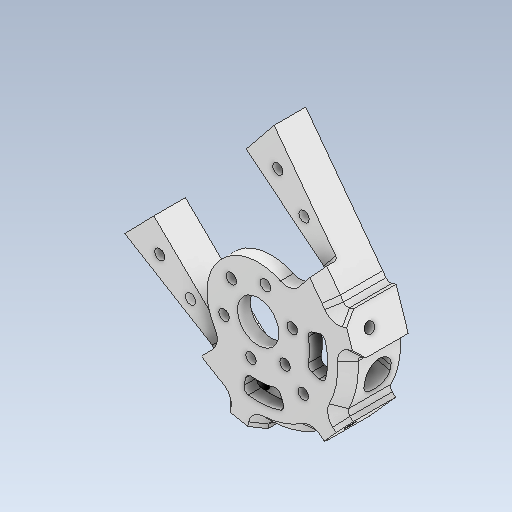
# Autodesk Inventor part: end_holder_1
Saved by Autodesk Inventor 2020 (Build 240168000, 168)
## iProperties
Created: 2020-08-12
Part Number: end_holder_1
Material: ABS Plastic
Document SubType Name: Modeling
Designer: psrobotics
Density: 1.06 g/cm^3
Appearance: Smooth - White
Author: psrobotics
Autodesk Inventor part; units mm, degrees
(part 1 of 2)
ref_plane "Work Plane1" through (0, 0, 1) normal (0, 0, 1) x (1, 0, 0)
sketch "Sketch1" plane through (0, 0, 1) normal (0, 0, 1) x (1, 0, 0)
  arc A0 (-18.1219, -29.9432) -> (28.0322, 20.957) centre (0, 0) ccw projected
  circle A1 centre (0, 0) radius 35
  circle A2 centre (0, 0) radius 26.3 projected
  circle A3 centre (0, 0) radius 29
  point P0 (0, 0)
  point P1 (28.0322, 20.957)
  dimension "d0" = 70
  dimension "d1" = 58
  constraints: 2 centre point, 2 coincident
  measures "d0" diameter of A1
  measures "d1" diameter of A3
ref_plane "Work Plane2" through (-254.295, -122.3855, -14.5) normal (0, 0, 1) x (0.9725249, -0.2327991, 0)
extrude "Extrusion1" add sketch "Sketch1" against normal up to surface (15.5 mm away) contours A1 A0
sketch "Sketch2" plane through (0, 0, 1) normal (0, 0, 1) x (1, 0, 0)
  circle A0 centre (-84.1417, 77.6558) radius 21 projected
  arc A1 (22.0166, 27.2079) -> (-24.4063, -25.0865) centre (0, 0) ccw projected
  line L0 (22.0166, 27.2079) -> (-113.9368, 137.2214) projected
  line L1 (-113.9368, 137.2214) -> (-123.7838, 141.4952) projected
  arc A2 (-156.6916, 110.1172) -> (-123.7838, 141.4952) centre (-169.0182, 155.9899) ccw projected
  line L2 (-156.6916, 110.1172) -> (-153.0652, 100.0837) projected
  line L3 (-153.0652, 100.0837) -> (-24.4063, -25.0865) projected
  circle A3 centre (-131.7071, 116.2642) radius 1.55 projected
  circle A4 centre (-150.4931, 104.7349) radius 1.55 projected
  circle A5 centre (-119.024, 134.2913) radius 1.55 projected
  circle A6 centre (0, 0) radius 35 projected
  circle A7 centre (0, 0) radius 29 projected
  line L4 (0, 0) -> (-24.4063, -25.0865)
  line L5 (0, 0) -> (22.0166, 27.2079)
  circle A8 centre (0, 0) radius 29 projected
  line L6 (-20.2223, -20.786) -> (-48.8927, 7.1069)
  line L7 (18.2423, 22.5437) -> (-12.8524, 47.7055)
  line L8 (-48.8927, 7.1069) -> (-53.0766, 2.8064)
  line L9 (-12.8524, 47.7055) -> (-9.0781, 52.3697)
  point P0 (0, 0)
  point P1 (3.0091, 34.8704)
  point P2 (-34.2679, -7.1213)
  dimension "d4" = 40
  dimension "d5" = 40
  constraints: 12 end point, 4 perpendicular, 4 point on line, 2 point on circle, 2 tangent
  measures "d4" distance of L6.start L6.end
  measures "d5" distance of L7.start L7.end
ref_plane "Work Plane3" through (-254.295, -122.3855, -14.5) normal (0, 0, 1) x (0.9725249, -0.2327991, 0)
extrude "Extrusion2" add sketch "Sketch2" against normal up to surface (15.5 mm away) contours A1 L7 L9 L0 | A1 L3 L8 L6
sketch "Sketch3" plane through (0, 0, 1) normal (0, 0, 1) x (1, 0, 0)
  arc A0 (-24.4063, -25.0865) -> (22.0166, 27.2079) centre (0, 0) ccw projected
  line L0 (22.0166, 27.2079) -> (-9.0781, 52.3697) projected
  line L1 (-9.0781, 52.3697) -> (-12.8524, 47.7055) projected
  line L2 (-12.8524, 47.7055) -> (3.0091, 34.8704) projected
  arc A1 (3.0091, 34.8704) -> (-34.2679, -7.1213) centre (0, 0) ccw projected
  line L3 (-34.2679, -7.1213) -> (-48.8927, 7.1069) projected
  line L4 (-48.8927, 7.1069) -> (-53.0766, 2.8064) projected
  line L5 (-53.0766, 2.8064) -> (-24.4063, -25.0865) projected
  circle A2 centre (0, 0) radius 29 projected
  line L6 (-34.2679, -7.1213) -> (-20.2223, -20.786)
  circle A3 centre (0, 0) radius 29 projected
  line L7 (3.0091, 34.8704) -> (18.2423, 22.5437)
  point P0 (0, 0)
  point P1 (-20.2223, -20.786)
  point P2 (18.2423, 22.5437)
  constraints: 4 end point, 2 point on circle, 2 tangent
ref_plane "Work Plane4" through (-254.295, -122.3855, -14.5) normal (0, 0, 1) x (0.9725249, -0.2327991, 0)
extrude "Extrusion3" cut sketch "Sketch3" against normal up to surface (15.5 mm away) contours A1 L7 A2 L6
sketch "Sketch4" plane through (0, 0, 1) normal (0, 0, 1) x (1, 0, 0)
  circle A0 centre (0, 0) radius 22 projected
  arc A1 (-134.634, 104.1043) -> (-137.4986, 97.7068) centre (-84.1417, 77.6558) ccw projected
  arc A2 (-140.9928, 97.2403) -> (-137.4986, 97.7068) centre (-139.3708, 98.4103) ccw projected
  arc A3 (-140.9928, 97.2403) -> (-143.7017, 100.0363) centre (-151.9418, 89.3428) ccw projected
  arc A4 (-143.3582, 103.4179) -> (-143.7017, 100.0363) centre (-142.481, 101.6206) ccw projected
  arc A5 (-143.3582, 103.4179) -> (-137.4838, 106.7169) centre (-169.0182, 155.9899) ccw projected
  arc A6 (-134.634, 104.1043) -> (-137.4838, 106.7169) centre (-136.4057, 105.0323) ccw projected
  arc A7 (-141.6259, 76.3096) -> (-139.9648, 63.8706) centre (-84.1417, 77.6558) ccw projected
  arc A8 (-143.4147, 62.0777) -> (-139.9648, 63.8706) centre (-141.9064, 63.3911) ccw projected
  line L0 (-143.4147, 62.0777) -> (-152.5393, 72.5562) projected
  arc A9 (-151.1485, 75.8661) -> (-152.5393, 72.5562) centre (-151.031, 73.8696) ccw projected
  arc A10 (-151.1485, 75.8661) -> (-144.6984, 77.9505) centre (-151.9418, 89.3428) ccw projected
  arc A11 (-141.6259, 76.3096) -> (-144.6984, 77.9505) centre (-143.6254, 76.2628) ccw projected
  arc A12 (-172.9205, 88.3973) -> (-165.3006, 73.1397) centre (-151.9418, 89.3428) ccw projected
  arc A13 (-170.8017, 90.4837) -> (-172.9205, 88.3973) centre (-170.9225, 88.4874) ccw projected
  line L1 (-170.8017, 90.4837) -> (-167.2842, 90.2709) projected
  arc A14 (-165.4097, 88.4124) -> (-167.2842, 90.2709) centre (-167.4049, 88.2746) ccw projected
  arc A15 (-165.4097, 88.4124) -> (-160.7764, 79.135) centre (-151.9418, 89.3428) ccw projected
  arc A16 (-160.4168, 76.52) -> (-160.7764, 79.135) centre (-162.0853, 77.6227) ccw projected
  line L2 (-160.4168, 76.52) -> (-162.3598, 73.5801) projected
  arc A17 (-165.3006, 73.1397) -> (-162.3598, 73.5801) centre (-164.0284, 74.6828) ccw projected
  arc A18 (-121.303, 49.7044) -> (-115.1167, 42.9745) centre (-84.1417, 77.6558) ccw projected
  arc A19 (-120.5392, 54.0239) -> (-121.303, 49.7044) centre (-118.9055, 51.5077) ccw projected
  line L3 (-120.5392, 54.0239) -> (-118.8576, 55.1157) projected
  arc A20 (-114.8324, 54.4108) -> (-118.8576, 55.1157) centre (-117.2239, 52.5995) ccw projected
  arc A21 (-114.8324, 54.4108) -> (-109.9637, 49.0993) centre (-84.1417, 77.6558) ccw projected
  arc A22 (-109.5035, 45.1747) -> (-109.9637, 49.0993) centre (-111.9758, 46.8741) ccw projected
  line L4 (-109.5035, 45.1747) -> (-110.6461, 43.5126) projected
  arc A23 (-115.1167, 42.9745) -> (-110.6461, 43.5126) centre (-113.1183, 45.212) ccw projected
  arc A24 (-66.7292, 111.9932) -> (-73.4322, 114.6363) centre (-84.1417, 77.6558) ccw projected
  arc A25 (-75.5321, 118.142) -> (-73.4322, 114.6363) centre (-72.5977, 117.5179) ccw projected
  line L5 (-75.5321, 118.142) -> (-74.177, 124.5142) projected
  arc A26 (-70.4364, 126.7798) -> (-74.177, 124.5142) centre (-71.2426, 123.8902) ccw projected
  arc A27 (-60.257, 122.7171) -> (-70.4364, 126.7798) centre (-84.1417, 77.6558) ccw projected
  arc A28 (-59.1897, 118.367) -> (-60.257, 122.7171) centre (-61.662, 120.0665) ccw projected
  line L6 (-59.1897, 118.367) -> (-62.9002, 112.9694) projected
  arc A29 (-66.7292, 111.9932) -> (-62.9002, 112.9694) centre (-65.3724, 114.6689) ccw projected
  arc A30 (-78.2994, 26.9916) -> (-67.6092, 29.4098) centre (-84.1417, 77.6558) ccw projected
  arc A31 (-81.6389, 29.8151) -> (-78.2994, 26.9916) centre (-78.643, 29.9718) ccw projected
  line L7 (-81.6389, 29.8151) -> (-81.9793, 36.3209) projected
  arc A32 (-79.3563, 39.4544) -> (-81.9793, 36.3209) centre (-78.9834, 36.4777) ccw projected
  arc A33 (-79.3563, 39.4544) -> (-72.322, 41.0151) centre (-84.1417, 77.6558) ccw projected
  arc A34 (-68.6931, 39.4512) -> (-72.322, 41.0151) centre (-71.401, 38.16) ccw projected
  line L8 (-68.6931, 39.4512) -> (-65.8738, 33.5391) projected
  arc A35 (-67.6092, 29.4098) -> (-65.8738, 33.5391) centre (-68.5817, 32.2478) ccw projected
  arc A36 (-122.585, 75.5668) -> (-121.5224, 68.4402) centre (-84.1417, 77.6558) ccw projected
  arc A37 (-123.5085, 64.8689) -> (-121.5224, 68.4402) centre (-124.4352, 67.7221) ccw projected
  line L9 (-123.5085, 64.8689) -> (-129.7045, 62.8563) projected
  arc A38 (-133.5369, 64.9629) -> (-129.7045, 62.8563) centre (-130.6313, 65.7096) ccw projected
  arc A39 (-135.1083, 75.8099) -> (-133.5369, 64.9629) centre (-84.1417, 77.6558) ccw projected
  arc A40 (-131.8746, 78.9093) -> (-135.1083, 75.8099) centre (-132.1102, 75.9185) ccw projected
  line L10 (-131.8746, 78.9093) -> (-125.3449, 78.3947) projected
  arc A41 (-122.585, 75.5668) -> (-125.3449, 78.3947) centre (-125.5805, 75.404) ccw projected
  arc A42 (-89.984, 128.3201) -> (-100.6741, 125.9019) centre (-84.1417, 77.6558) ccw projected
  arc A43 (-86.6444, 125.4966) -> (-89.984, 128.3201) centre (-89.6403, 125.3399) ccw projected
  line L11 (-86.6444, 125.4966) -> (-86.3041, 118.9907) projected
  arc A44 (-88.9271, 115.8573) -> (-86.3041, 118.9907) centre (-89.3, 118.834) ccw projected
  arc A45 (-88.9271, 115.8573) -> (-95.9613, 114.2966) centre (-84.1417, 77.6558) ccw projected
  arc A46 (-99.5902, 115.8604) -> (-95.9613, 114.2966) centre (-96.8824, 117.1517) ccw projected
  line L12 (-99.5902, 115.8604) -> (-102.4095, 121.7726) projected
  arc A47 (-100.6741, 125.9019) -> (-102.4095, 121.7726) centre (-99.7016, 123.0639) ccw projected
  arc A48 (-41.3543, 59.4489) -> (-38.6192, 68.1713) centre (-84.1417, 77.6558) ccw projected
  arc A49 (-45.477, 57.9506) -> (-41.3543, 59.4489) centre (-44.1148, 60.6235) ccw projected
  line L13 (-45.477, 57.9506) -> (-47.2634, 58.8611) projected
  arc A50 (-48.6656, 62.6994) -> (-47.2634, 58.8611) centre (-45.9012, 61.534) ccw projected
  arc A51 (-48.6656, 62.6994) -> (-46.5, 69.5716) centre (-84.1417, 77.6558) ccw projected
  arc A52 (-43.3312, 71.9324) -> (-46.5, 69.5716) centre (-43.5669, 68.9417) ccw projected
  line L14 (-43.3312, 71.9324) -> (-41.3205, 71.7739) projected
  arc A53 (-38.6192, 68.1713) -> (-41.3205, 71.7739) centre (-41.5561, 68.7832) ccw projected
  line L15 (-106.5258, 40.6801) -> (-105.3832, 42.3423) projected
  arc A54 (-101.5541, 43.3185) -> (-105.3832, 42.3423) centre (-102.911, 40.6428) ccw projected
  arc A55 (-101.5541, 43.3185) -> (-94.8511, 40.6753) centre (-84.1417, 77.6558) ccw projected
  arc A56 (-92.7512, 37.1697) -> (-94.8511, 40.6753) centre (-95.6856, 37.7937) ccw projected
  line L16 (-92.7512, 37.1697) -> (-93.1683, 35.2086) projected
  arc A57 (-96.9276, 32.9482) -> (-93.1683, 35.2086) centre (-96.1027, 35.8326) ccw projected
  arc A58 (-105.4268, 36.3134) -> (-96.9276, 32.9482) centre (-84.1417, 77.6558) ccw projected
  arc A59 (-106.5258, 40.6801) -> (-105.4268, 36.3134) centre (-104.0535, 38.9807) ccw projected
  arc A60 (-58.7798, 110.137) -> (-58.3197, 106.2124) centre (-56.3076, 108.4375) ccw projected
  line L17 (-58.7798, 110.137) -> (-55.0694, 115.5346) projected
  arc A61 (-50.6256, 116.0964) -> (-55.0694, 115.5346) centre (-52.5971, 113.8352) ccw projected
  arc A62 (-43.1863, 108.0475) -> (-50.6256, 116.0964) centre (-84.1417, 77.6558) ccw projected
  arc A63 (-43.9617, 103.7436) -> (-43.1863, 108.0475) centre (-45.5954, 106.2598) ccw projected
  line L18 (-43.9617, 103.7436) -> (-49.4258, 100.196) projected
  arc A64 (-53.451, 100.9008) -> (-49.4258, 100.196) centre (-51.0595, 102.7121) ccw projected
  arc A65 (-53.451, 100.9008) -> (-58.3197, 106.2124) centre (-84.1417, 77.6558) ccw projected
  line L19 (-61.3607, 35.6912) -> (-64.18, 41.6034) projected
  arc A66 (-63.1109, 45.4075) -> (-64.18, 41.6034) centre (-61.4721, 42.8946) ccw projected
  arc A67 (-63.1109, 45.4075) -> (-57.4703, 49.8909) centre (-84.1417, 77.6558) ccw projected
  arc A68 (-53.3844, 49.9567) -> (-57.4703, 49.8909) centre (-55.392, 47.7274) ccw projected
  line L20 (-53.3844, 49.9567) -> (-48.5435, 45.597) projected
  arc A69 (-48.4517, 41.2248) -> (-48.5435, 45.597) centre (-50.5511, 43.3678) ccw projected
  arc A70 (-57.0598, 34.4404) -> (-48.4517, 41.2248) centre (-84.1417, 77.6558) ccw projected
  arc A71 (-61.3607, 35.6912) -> (-57.0598, 34.4404) centre (-58.6528, 36.9825) ccw projected
  arc A72 (-124.9521, 83.3793) -> (-121.7833, 85.7401) centre (-124.7165, 86.37) ccw projected
  line L21 (-124.9521, 83.3793) -> (-131.4818, 83.8938) projected
  arc A73 (-134.1902, 87.4613) -> (-131.4818, 83.8938) centre (-131.2461, 86.8845) ccw projected
  arc A74 (-130.9394, 97.9284) -> (-134.1902, 87.4613) centre (-84.1417, 77.6558) ccw projected
  arc A75 (-126.8243, 99.4088) -> (-130.9394, 97.9284) centre (-128.1866, 96.7359) ccw projected
  line L22 (-126.8243, 99.4088) -> (-121.0199, 96.4506) projected
  arc A76 (-119.6178, 92.6123) -> (-121.0199, 96.4506) centre (-122.3822, 93.7777) ccw projected
  arc A77 (-119.6178, 92.6123) -> (-121.7833, 85.7401) centre (-84.1417, 77.6558) ccw projected
  line L23 (-106.9226, 119.6204) -> (-104.1034, 113.7083) projected
  arc A78 (-105.1725, 109.9042) -> (-104.1034, 113.7083) centre (-106.8112, 112.417) ccw projected
  arc A79 (-105.1725, 109.9042) -> (-110.813, 105.4207) centre (-84.1417, 77.6558) ccw projected
  arc A80 (-114.8989, 105.355) -> (-110.813, 105.4207) centre (-112.8913, 107.5842) ccw projected
  line L24 (-114.8989, 105.355) -> (-119.7399, 109.7147) projected
  arc A81 (-119.8317, 114.0869) -> (-119.7399, 109.7147) centre (-117.7323, 111.9439) ccw projected
  arc A82 (-111.2236, 120.8712) -> (-119.8317, 114.0869) centre (-84.1417, 77.6558) ccw projected
  arc A83 (-106.9226, 119.6204) -> (-111.2236, 120.8712) centre (-109.6305, 118.3292) ccw projected
  line L25 (-40.9277, 76.7585) -> (-42.9385, 76.9169) projected
  arc A84 (-45.6984, 79.7449) -> (-42.9385, 76.9169) centre (-42.7028, 79.9077) ccw projected
  arc A85 (-45.6984, 79.7449) -> (-46.7609, 86.8714) centre (-84.1417, 77.6558) ccw projected
  arc A86 (-44.7749, 90.4428) -> (-46.7609, 86.8714) centre (-43.8481, 87.5895) ccw projected
  line L26 (-44.7749, 90.4428) -> (-42.868, 91.0622) projected
  arc A87 (-39.0308, 88.9367) -> (-42.868, 91.0622) centre (-41.9412, 88.2089) ccw projected
  arc A88 (-37.6955, 79.8936) -> (-39.0308, 88.9367) centre (-84.1417, 77.6558) ccw projected
  arc A89 (-40.9277, 76.7585) -> (-37.6955, 79.8936) centre (-40.6921, 79.7492) ccw projected
  circle A90 centre (-150.4931, 104.7349) radius 2.1 projected
  circle A91 centre (-131.7071, 116.2642) radius 2.1 projected
  circle A92 centre (-172.3092, 101.5894) radius 2.1 projected
  circle A93 centre (-119.024, 134.2913) radius 2.1 projected
  circle A94 centre (-151.9418, 89.3428) radius 8 projected
  line L27 (-121.4797, 140.4951) -> (-109.1576, 143.9934) projected
  arc A95 (-172.0375, 106.0811) -> (-121.4797, 140.4951) centre (-169.0182, 155.9899) ccw projected
  line L28 (-172.0375, 106.0811) -> (-180.4523, 106.5902) projected
  line L29 (-180.4523, 106.5902) -> (-181.871, 83.1388) projected
  line L30 (-181.871, 83.1388) -> (-178.1654, 82.9146) projected
  arc A96 (-178.1654, 82.9146) -> (-161.4844, 64.0853) centre (-151.9418, 89.3428) ccw projected
  line L31 (-161.4844, 64.0853) -> (-161.7085, 60.3797) projected
  line L32 (-161.7085, 60.3797) -> (-153.7231, 59.8966) projected
  line L33 (-153.7231, 59.8966) -> (-113.0893, 33.8576) projected
  line L34 (-113.0893, 33.8576) -> (-116.9889, 27.9573) projected
  line L35 (-116.9889, 27.9573) -> (-102.5081, 21.1281) projected
  line L36 (-102.5081, 21.1281) -> (-18.1219, -29.9432) projected
  arc A97 (-18.1219, -29.9432) -> (28.0322, 20.957) centre (0, 0) ccw projected
  line L37 (28.0322, 20.957) -> (-27.0336, 94.6133) projected
  line L38 (-27.0336, 94.6133) -> (-33.7368, 109.1529) projected
  arc A98 (-33.7368, 109.1529) -> (-36.6738, 113.4261) centre (-84.1417, 77.6558) ccw projected
  line L39 (-36.6738, 113.4261) -> (-37.4491, 112.8418) projected
  arc A99 (-40.2079, 113.1815) -> (-37.4491, 112.8418) centre (-38.6527, 114.4391) ccw projected
  arc A100 (-40.2079, 113.1815) -> (-46.2045, 119.5249) centre (-84.1417, 77.6558) ccw projected
  arc A101 (-46.3887, 122.2985) -> (-46.2045, 119.5249) centre (-44.8616, 121.007) ccw projected
  line L40 (-46.3887, 122.2985) -> (-45.5261, 123.3186) projected
  arc A102 (-45.5261, 123.3186) -> (-50.5107, 127.1049) centre (-84.1417, 77.6558) ccw projected
  line L41 (-50.5107, 127.1049) -> (-61.0603, 132.8238) projected
  arc A103 (-61.0603, 132.8238) -> (-66.9533, 134.9342) centre (-84.1417, 77.6558) ccw projected
  line L42 (-66.9533, 134.9342) -> (-67.3373, 133.6546) projected
  arc A104 (-69.762, 132.2953) -> (-67.3373, 133.6546) centre (-69.2529, 134.2295) ccw projected
  arc A105 (-69.762, 132.2953) -> (-78.35, 133.8582) centre (-84.1417, 77.6558) ccw projected
  arc A106 (-80.1403, 135.9846) -> (-78.35, 133.8582) centre (-78.145, 135.8477) ccw projected
  line L43 (-80.1403, 135.9846) -> (-80.0739, 136.9531) projected
  arc A107 (-80.0739, 136.9531) -> (-85.2575, 137.082) centre (-84.1417, 77.6558) ccw projected
  line L44 (-85.2575, 137.082) -> (-101.0991, 134.7639) projected
  line L45 (-101.0991, 134.7639) -> (-109.1576, 143.9934) projected
  circle A108 centre (-178.1359, 86.9201) radius 1.5 projected
  circle A109 centre (-100.501, 24.1648) radius 1.5 projected
  circle A110 centre (-64.7276, 24.8072) radius 1.5 projected
  circle A111 centre (-37.2263, 108.1168) radius 1.5 projected
  circle A112 centre (-65.0433, 130.6194) radius 1.5 projected
  circle A113 centre (-84.2213, 133.5925) radius 1.5 projected
  circle A114 centre (-50.1841, 122.5643) radius 1.5 projected
  circle A115 centre (-48.1253, 34.857) radius 1.5 projected
  circle A116 centre (-81.2881, 21.4264) radius 1.5 projected
  circle A117 centre (-157.5045, 63.6318) radius 1.5 projected
  circle A118 centre (-84.1417, 77.6558) radius 32.5 projected
  line L46 (-20.2223, -20.786) -> (-48.8927, 7.1069) projected
  line L47 (-48.8927, 7.1069) -> (-53.0766, 2.8064) projected
  line L48 (-53.0766, 2.8064) -> (-24.4063, -25.0865) projected
  arc A119 (-24.4063, -25.0865) -> (22.0166, 27.2079) centre (0, 0) ccw projected
  line L49 (22.0166, 27.2079) -> (-9.0781, 52.3697) projected
  line L50 (-9.0781, 52.3697) -> (-12.8524, 47.7055) projected
  line L51 (-12.8524, 47.7055) -> (18.2423, 22.5437) projected
  arc A120 (-20.2223, -20.786) -> (18.2423, 22.5437) centre (0, 0) ccw projected
  line L52 (-12.8524, 47.7055) -> (-9.0781, 52.3697) projected
  line L53 (-9.0781, 52.3697) -> (-1.9955, 61.1223)
  line L54 (-53.0766, 2.8064) -> (-60.1765, -4.4914)
  line L55 (-48.8927, 7.1069) -> (-53.0766, 2.8064) projected
  circle A121 centre (9.6755, 36.1764) radius 2 projected
  circle A122 centre (-34.5876, -13.7627) radius 2 projected
  circle A123 centre (-0.5842, 47.1189) radius 2 projected
  circle A124 centre (-46.5558, -4.7204) radius 2 projected
  point P0 (0, 0)
  point P1 (-18.1219, -29.9432)
  point P2 (28.0322, 20.957)
  constraints: 4 end point, 3 point on line, 1 collinear
extrude "Extrusion4" add sketch "Sketch4" against normal up to surface (15.5 mm away) contours L54 L48 A124 A122 A119 L36 | A119 L49 A121 A123 L53 L37 | L48 A124 | A122 L48 | L49 A121 | A123 L49 picked at (-46.2816, -4.9711) picked at (-35.4873, -14.8787) picked at (9.9892, 37.2529) picked at (-0.3031, 46.513)
ref_plane "Work Plane5" through (-227.4633, -98.5759, -2.2) normal (0, 0, -1) x (0.2327991, 0.9725249, 0)
sketch "Sketch5" plane through (0, 0, 1) normal (0, 0, 1) x (1, 0, 0)
  line L0 (-20.2223, -20.786) -> (-48.8927, 7.1069) projected
  line L1 (-48.8927, 7.1069) -> (-60.1765, -4.4914) projected
  line L2 (-60.1765, -4.4914) -> (-18.1219, -29.9432) projected
  arc A0 (-18.1219, -29.9432) -> (28.0322, 20.957) centre (0, 0) ccw projected
  line L3 (28.0322, 20.957) -> (-1.9955, 61.1223) projected
  line L4 (-1.9955, 61.1223) -> (-12.8524, 47.7055) projected
  line L5 (-12.8524, 47.7055) -> (18.2423, 22.5437) projected
  arc A1 (-20.2223, -20.786) -> (18.2423, 22.5437) centre (0, 0) ccw projected
  line L6 (-60.1765, -4.4914) -> (-18.1219, -29.9432) projected
  line L7 (0, 0) -> (-18.1219, -29.9432)
  line L8 (28.0322, 20.957) -> (-1.9955, 61.1223) projected
  line L9 (0, 0) -> (28.0322, 20.957)
  point P0 (0, 0)
  point P1 (23.2267, 17.3644)
  point P2 (-15.0153, -24.8101)
  constraints: 4 end point, 2 perpendicular
extrude "Extrusion5" cut sketch "Sketch5" against normal up to surface (3.2 mm away) contours A1 L7 L2 L1 L0 | A1 L5 L4 L3 L9
sketch "Sketch8" plane through (-60.1765, -4.4914, -2.2) normal (0, 0, 1) x (0.8555205, -0.517769, 0)
  circle A0 centre (38.7033, 70.9593) radius 2 projected
  circle A1 centre (26.6922, 5.3173) radius 2 projected
  circle A2 centre (24.2602, 75.0087) radius 2 projected
  circle A3 centre (11.7714, 6.8564) radius 2 projected
  circle A4 centre (49.1567, 35) radius 22 projected
  arc A5 (-119.9275, 54.354) -> (-119.0657, 47.3976) centre (-63.036, 57.8702) ccw projected
  arc A6 (-121.8136, 45.1894) -> (-119.0657, 47.3976) centre (-121.0316, 47.0302) ccw projected
  arc A7 (-121.8136, 45.1894) -> (-125.5788, 46.1788) centre (-127.0915, 32.7639) ccw projected
  arc A8 (-127.0358, 49.2497) -> (-125.5788, 46.1788) centre (-125.3547, 48.1662) ccw projected
  arc A9 (-127.0358, 49.2497) -> (-123.7182, 55.1136) centre (-176.2086, 80.9402) ccw projected
  arc A10 (-119.9275, 54.354) -> (-123.7182, 55.1136) centre (-121.9237, 54.2307) ccw projected
  arc A11 (-111.5179, 26.9549) -> (-103.6562, 17.1732) centre (-63.036, 57.8702) ccw projected
  arc A12 (-105.6794, 13.853) -> (-103.6562, 17.1732) centre (-105.0691, 15.7576) ccw projected
  line L0 (-105.6794, 13.853) -> (-118.9111, 18.0932) projected
  arc A13 (-119.4351, 21.645) -> (-118.9111, 18.0932) centre (-118.3008, 19.9978) ccw projected
  arc A14 (-119.4351, 21.645) -> (-114.9962, 26.7679) centre (-127.0915, 32.7639) ccw projected
  arc A15 (-111.5179, 26.9549) -> (-114.9962, 26.7679) centre (-113.2042, 25.8796) ccw projected
  arc A16 (-144.5497, 21.0929) -> (-130.1308, 11.985) centre (-127.0915, 32.7639) ccw projected
  arc A17 (-143.8174, 23.9748) -> (-144.5497, 21.0929) centre (-142.887, 22.2044) ccw projected
  line L1 (-143.8174, 23.9748) -> (-140.6978, 25.6141) projected
  arc A18 (-138.1319, 24.9946) -> (-140.6978, 25.6141) centre (-139.7675, 23.8436) ccw projected
  arc A19 (-138.1319, 24.9946) -> (-129.3645, 19.4566) centre (-127.0915, 32.7639) ccw projected
  arc A20 (-127.7028, 17.4056) -> (-129.3645, 19.4566) centre (-129.7012, 17.4851) ccw projected
  line L2 (-127.7028, 17.4056) -> (-127.843, 13.8844) projected
  arc A21 (-130.1308, 11.985) -> (-127.843, 13.8844) centre (-129.8414, 13.9639) ccw projected
  arc A22 (-80.3559, 14.7162) -> (-71.5789, 12.1617) centre (-63.036, 57.8702) ccw projected
  arc A23 (-81.9389, 18.8071) -> (-80.3559, 14.7162) centre (-79.2385, 17.5003) ccw projected
  line L3 (-81.9389, 18.8071) -> (-81.0656, 20.6119) projected
  arc A24 (-77.257, 22.0929) -> (-81.0656, 20.6119) centre (-78.3651, 19.3051) ccw projected
  arc A25 (-77.257, 22.0929) -> (-70.3416, 20.0697) centre (-63.036, 57.8702) ccw projected
  arc A26 (-67.9159, 16.9503) -> (-70.3416, 20.0697) centre (-70.9108, 17.1242) ccw projected
  line L4 (-67.9159, 16.9503) -> (-68.0328, 14.9368) projected
  arc A27 (-71.5789, 12.1617) -> (-68.0328, 14.9368) centre (-71.0277, 15.1106) ccw projected
  arc A28 (-65.9181, 96.2622) -> (-73.0212, 95.0528) centre (-63.036, 57.8702) ccw projected
  arc A29 (-76.6328, 96.9647) -> (-73.0212, 95.0528) centre (-73.7993, 97.9502) ccw projected
  line L5 (-76.6328, 96.9647) -> (-78.7729, 103.1179) projected
  arc A30 (-76.7458, 106.9929) -> (-78.7729, 103.1179) centre (-75.9393, 104.1034) ccw projected
  arc A31 (-65.9335, 108.7878) -> (-76.7458, 106.9929) centre (-63.036, 57.8702) ccw projected
  arc A32 (-62.7681, 105.6188) -> (-65.9335, 108.7878) centre (-65.7631, 105.7927) ccw projected
  line L6 (-62.7681, 105.6188) -> (-63.1477, 99.0799) projected
  arc A33 (-65.9181, 96.2622) -> (-63.1477, 99.0799) centre (-66.1427, 99.2538) ccw projected
  arc A34 (-31.8054, 17.5509) -> (-23.9119, 25.1547) centre (-63.036, 57.8702) ccw projected
  arc A35 (-36.1244, 18.2373) -> (-31.8054, 17.5509) centre (-33.6425, 19.9226) ccw projected
  line L7 (-36.1244, 18.2373) -> (-39.7841, 23.627) projected
  arc A36 (-39.1625, 27.6658) -> (-39.7841, 23.627) centre (-37.3022, 25.3122) ccw projected
  arc A37 (-39.1625, 27.6658) -> (-33.9526, 32.6432) centre (-63.036, 57.8702) ccw projected
  arc A38 (-30.0383, 33.1842) -> (-33.9526, 32.6432) centre (-31.6864, 30.6774) ccw projected
  line L8 (-30.0383, 33.1842) -> (-24.5652, 29.586) projected
  arc A39 (-23.9119, 25.1547) -> (-24.5652, 29.586) centre (-26.2133, 27.0792) ccw projected
  arc A40 (-94.8434, 36.1783) -> (-90.2445, 30.6315) centre (-63.036, 57.8702) ccw projected
  arc A41 (-90.0944, 26.5478) -> (-90.2445, 30.6315) centre (-92.3646, 28.509) ccw projected
  line L9 (-90.0944, 26.5478) -> (-94.3532, 21.6179) projected
  arc A42 (-98.7226, 21.4358) -> (-94.3532, 21.6179) centre (-96.6234, 23.579) ccw projected
  arc A43 (-105.6832, 29.9021) -> (-98.7226, 21.4358) centre (-63.036, 57.8702) ccw projected
  arc A44 (-104.5215, 34.2279) -> (-105.6832, 29.9021) centre (-103.1746, 31.5473) ccw projected
  line L10 (-104.5215, 34.2279) -> (-98.6688, 37.1686) projected
  arc A45 (-94.8434, 36.1783) -> (-98.6688, 37.1686) centre (-97.3219, 34.488) ccw projected
  arc A46 (-94.2666, 98.1896) -> (-102.1602, 90.5857) centre (-63.036, 57.8702) ccw projected
  arc A47 (-89.9476, 97.5031) -> (-94.2666, 98.1896) centre (-92.4295, 95.8178) ccw projected
  line L11 (-89.9476, 97.5031) -> (-86.2879, 92.1135) projected
  arc A48 (-86.9095, 88.0746) -> (-86.2879, 92.1135) centre (-88.7698, 90.4282) ccw projected
  arc A49 (-86.9095, 88.0746) -> (-92.1194, 83.0973) centre (-63.036, 57.8702) ccw projected
  arc A50 (-96.0337, 82.5562) -> (-92.1194, 83.0973) centre (-94.3857, 85.063) ccw projected
  line L12 (-96.0337, 82.5562) -> (-101.5068, 86.1545) projected
  arc A51 (-102.1602, 90.5857) -> (-101.5068, 86.1545) centre (-99.8587, 88.6612) ccw projected
  arc A52 (-17.0036, 64.4478) -> (-19.1798, 73.3261) centre (-63.036, 57.8702) ccw projected
  arc A53 (-19.7549, 61.0314) -> (-17.0036, 64.4478) centre (-19.9734, 64.0234) ccw projected
  line L13 (-19.7549, 61.0314) -> (-21.7546, 60.8853) projected
  arc A54 (-24.9415, 63.4431) -> (-21.7546, 60.8853) centre (-21.9731, 63.8774) ccw projected
  arc A55 (-24.9415, 63.4431) -> (-26.647, 70.4437) centre (-63.036, 57.8702) ccw projected
  arc A56 (-25.1584, 74.1041) -> (-26.647, 70.4437) centre (-23.8115, 71.4234) ccw projected
  line L14 (-25.1584, 74.1041) -> (-23.3562, 75.0096) projected
  arc A57 (-19.1798, 73.3261) -> (-23.3562, 75.0096) centre (-22.0093, 72.329) ccw projected
  line L15 (-63.0412, 14.647) -> (-62.9243, 16.6605) projected
  arc A58 (-60.1539, 19.4782) -> (-62.9243, 16.6605) centre (-59.9293, 16.4867) ccw projected
  arc A59 (-60.1539, 19.4782) -> (-53.0508, 20.6876) centre (-63.036, 57.8702) ccw projected
  arc A60 (-49.4392, 18.7758) -> (-53.0508, 20.6876) centre (-52.2727, 17.7903) ccw projected
  line L16 (-49.4392, 18.7758) -> (-48.7806, 16.882) projected
  arc A61 (-50.8264, 13.0018) -> (-48.7806, 16.882) centre (-51.6141, 15.8965) ccw projected
  arc A62 (-59.84, 11.4802) -> (-50.8264, 13.0018) centre (-63.036, 57.8702) ccw projected
  arc A63 (-63.0412, 14.647) -> (-59.84, 11.4802) centre (-60.0462, 14.4731) ccw projected
  arc A64 (-58.1561, 98.7901) -> (-55.7305, 95.6707) centre (-55.1612, 98.6162) ccw projected
  line L17 (-58.1561, 98.7901) -> (-57.7765, 105.329) projected
  arc A65 (-54.2657, 108.1104) -> (-57.7765, 105.329) centre (-54.7816, 105.1551) ccw projected
  arc A66 (-43.7337, 105.0764) -> (-54.2657, 108.1104) centre (-63.036, 57.8702) ccw projected
  arc A67 (-42.1687, 100.9928) -> (-43.7337, 105.0764) centre (-44.8691, 102.2995) ccw projected
  line L18 (-42.1687, 100.9928) -> (-45.0064, 95.1286) projected
  arc A68 (-48.815, 93.6475) -> (-45.0064, 95.1286) centre (-47.7069, 96.4353) ccw projected
  arc A69 (-48.815, 93.6475) -> (-55.7305, 95.6707) centre (-63.036, 57.8702) ccw projected
  line L19 (-21.8185, 33.7639) -> (-27.2915, 37.3621) projected
  arc A70 (-28.3465, 41.1702) -> (-27.2915, 37.3621) centre (-25.6435, 39.8689) ccw projected
  arc A71 (-28.3465, 41.1702) -> (-25.8423, 47.9264) centre (-63.036, 57.8702) ccw projected
  arc A72 (-22.3808, 50.0982) -> (-25.8423, 47.9264) centre (-22.9441, 47.1515) ccw projected
  line L20 (-22.3808, 50.0982) -> (-15.982, 48.8749) projected
  arc A73 (-13.6396, 45.1819) -> (-15.982, 48.8749) centre (-16.5453, 45.9282) ccw projected
  arc A74 (-17.4913, 34.9207) -> (-13.6396, 45.1819) centre (-63.036, 57.8702) ccw projected
  arc A75 (-21.8185, 33.7639) -> (-17.4913, 34.9207) centre (-20.1704, 36.2707) ccw projected
  arc A76 (-100.9136, 41.6364) -> (-99.425, 45.2968) centre (-102.2605, 44.317) ccw projected
  line L21 (-100.9136, 41.6364) -> (-106.7663, 38.6957) projected
  arc A77 (-110.9305, 40.3455) -> (-106.7663, 38.6957) centre (-108.1132, 41.3763) ccw projected
  arc A78 (-113.5689, 50.9834) -> (-110.9305, 40.3455) centre (-63.036, 57.8702) ccw projected
  arc A79 (-110.8149, 54.3805) -> (-113.5689, 50.9834) centre (-110.5964, 51.3885) ccw projected
  line L22 (-110.8149, 54.3805) -> (-104.3175, 54.8551) projected
  arc A80 (-101.1305, 52.2973) -> (-104.3175, 54.8551) centre (-104.0989, 51.8631) ccw projected
  arc A81 (-101.1305, 52.2973) -> (-99.425, 45.2968) centre (-63.036, 57.8702) ccw projected
  line L23 (-104.2536, 81.9765) -> (-98.7805, 78.3783) projected
  arc A82 (-97.7255, 74.5702) -> (-98.7805, 78.3783) centre (-100.4286, 75.8715) ccw projected
  arc A83 (-97.7255, 74.5702) -> (-100.2297, 67.8141) centre (-63.036, 57.8702) ccw projected
  arc A84 (-103.6912, 65.6423) -> (-100.2297, 67.8141) centre (-103.1279, 68.5889) ccw projected
  line L24 (-103.6912, 65.6423) -> (-110.0901, 66.8655) projected
  arc A85 (-112.4324, 70.5586) -> (-110.0901, 66.8655) centre (-109.5268, 69.8122) ccw projected
  arc A86 (-108.5807, 80.8197) -> (-112.4324, 70.5586) centre (-63.036, 57.8702) ccw projected
  arc A87 (-104.2536, 81.9765) -> (-108.5807, 80.8197) centre (-105.9016, 79.4698) ccw projected
  line L25 (-25.601, 79.4774) -> (-27.4032, 78.5718) projected
  arc A88 (-31.2286, 79.5622) -> (-27.4032, 78.5718) centre (-28.7501, 81.2525) ccw projected
  arc A89 (-31.2286, 79.5622) -> (-35.8275, 85.109) centre (-63.036, 57.8702) ccw projected
  arc A90 (-35.9776, 89.1926) -> (-35.8275, 85.109) centre (-33.7074, 87.2315) ccw projected
  line L26 (-35.9776, 89.1926) -> (-34.6669, 90.7099) projected
  arc A91 (-30.2836, 90.8783) -> (-34.6669, 90.7099) centre (-32.3967, 88.7487) ccw projected
  arc A92 (-24.459, 83.833) -> (-30.2836, 90.8783) centre (-63.036, 57.8702) ccw projected
  arc A93 (-25.601, 79.4774) -> (-24.459, 83.833) centre (-26.9479, 82.158) ccw projected
  circle A94 centre (-133.8217, 46.6822) radius 2.1 projected
  circle A95 centre (-123.7194, 66.2726) radius 2.1 projected
  circle A96 centre (-150.8572, 32.6954) radius 2.1 projected
  circle A97 centre (-122.2026, 88.262) radius 2.1 projected
  circle A98 centre (-127.0915, 32.7639) radius 8 projected
  line L27 (-127.5157, 92.2981) -> (-118.7852, 101.6709) projected
  arc A99 (-152.9504, 36.6789) -> (-127.5157, 92.2981) centre (-176.2086, 80.9402) ccw projected
  line L28 (-152.9504, 36.6789) -> (-160.4131, 32.7575) projected
  line L29 (-160.4131, 32.7575) -> (-149.4844, 11.9597) projected
  line L30 (-149.4844, 11.9597) -> (-146.1981, 13.6866) projected
  arc A100 (-146.1981, 13.6866) -> (-122.1779, 6.2147) centre (-127.0915, 32.7639) ccw projected
  line L31 (-122.1779, 6.2147) -> (-120.451, 2.9284) projected
  line L32 (-120.451, 2.9284) -> (-113.3692, 6.6497) projected
  line L33 (-113.3692, 6.6497) -> (-65.1239, 5.4117) projected
  line L34 (-65.1239, 5.4117) -> (-65.4052, -1.6552) projected
  line L35 (-65.4052, -1.6552) -> (-49.4806, 0) projected
  line L36 (-49.4806, 0) -> (49.1567, 0) projected
  arc A101 (49.1567, 0) -> (62.2879, 67.4433) centre (49.1567, 35) ccw projected
  line L37 (62.2879, 67.4433) -> (-22.9589, 101.9465) projected
  line L38 (-22.9589, 101.9465) -> (-36.2218, 110.9146) projected
  arc A102 (-36.2218, 110.9146) -> (-40.947, 113.0498) centre (-63.036, 57.8702) ccw projected
  line L39 (-40.947, 113.0498) -> (-41.3078, 112.1485) projected
  arc A103 (-43.8439, 111.0107) -> (-41.3078, 112.1485) centre (-43.1645, 112.8918) ccw projected
  arc A104 (-43.8439, 111.0107) -> (-52.2585, 113.3328) centre (-63.036, 57.8702) ccw projected
  arc A105 (-53.8522, 115.6102) -> (-52.2585, 113.3328) centre (-51.877, 115.2961) ccw projected
  line L40 (-53.8522, 115.6102) -> (-53.6423, 116.9296) projected
  arc A106 (-53.6423, 116.9296) -> (-59.8672, 117.588) centre (-63.036, 57.8702) ccw projected
  line L41 (-59.8672, 117.588) -> (-71.8537, 117.0183) projected
  arc A107 (-71.8537, 117.0183) -> (-77.988, 115.7726) centre (-63.036, 57.8702) ccw projected
  line L42 (-77.988, 115.7726) -> (-77.654, 114.4791) projected
  arc A108 (-79.0245, 112.0608) -> (-77.654, 114.4791) centre (-79.5905, 113.979) ccw projected
  arc A109 (-79.0245, 112.0608) -> (-87.181, 108.9512) centre (-63.036, 57.8702) ccw projected
  arc A110 (-89.8136, 109.8434) -> (-87.181, 108.9512) centre (-88.0357, 110.7594) ccw projected
  line L43 (-89.8136, 109.8434) -> (-90.2582, 110.7064) projected
  arc A111 (-90.2582, 110.7064) -> (-94.7596, 108.1328) centre (-63.036, 57.8702) ccw projected
  line L44 (-94.7596, 108.1328) -> (-107.1123, 97.9473) projected
  line L45 (-107.1123, 97.9473) -> (-118.7852, 101.6709) projected
  circle A112 centre (-148.2467, 17.1287) radius 1.5 projected
  circle A113 centre (-49.3358, 3.6372) radius 1.5 projected
  circle A114 centre (-19.0635, 22.7091) radius 1.5 projected
  circle A115 centre (-38.6707, 108.2215) radius 1.5 projected
  circle A116 centre (-74.1198, 113.0702) radius 1.5 projected
  circle A117 centre (-92.0664, 105.684) radius 1.5 projected
  circle A118 centre (-57.2368, 113.8725) radius 1.5 projected
  circle A119 centre (-10.0634, 39.9031) radius 1.5 projected
  circle A120 centre (-31.4809, 11.2423) radius 1.5 projected
  circle A121 centre (-118.5382, 7.8874) radius 1.5 projected
  circle A122 centre (-63.036, 57.8702) radius 32.5 projected
  point P0 (49.1567, 35)
extrude "Extrusion7" cut sketch "Sketch8" against normal blind 14 contours A0 | A1 | A2 | A3
sketch "Sketch9" plane through (0, 0, 1) normal (0, 0, 1) x (1, 0, 0)
  circle A0 centre (0, 0) radius 8.075
  circle A1 centre (0, 0) radius 20
  line L0 (28.0322, 20.957) -> (23.2267, 17.3644) projected
  arc A2 (-15.0153, -24.8101) -> (23.2267, 17.3644) centre (0, 0) ccw projected
  line L1 (-15.0153, -24.8101) -> (-18.1219, -29.9432) projected
  arc A3 (-18.1219, -29.9432) -> (28.0322, 20.957) centre (0, 0) ccw projected
  line L2 (23.2267, 17.3644) -> (28.0322, 20.957) projected
  line L3 (0, 0) -> (28.0322, 20.957)
  line L4 (-18.1219, -29.9432) -> (-15.0153, -24.8101) projected
  line L5 (0, 0) -> (-18.1219, -29.9432)
  point P0 (16.0184, 11.9754)
  point P1 (-10.3554, -17.1104)
  point P2 (-15.0153, -24.8101)
  point P3 (23.2267, 17.3644)
  dimension "d26" = 16.15
  dimension "d27" = 40
  constraints: 4 end point, 2 centre point, 2 coincident, 2 collinear
  measures "d26" diameter of A0
  measures "d27" diameter of A1
extrude "Extrusion8" add sketch "Sketch9" along normal blind 5 contours A0 L3 A1 L5 | A0 L5 A1 L3 | L3 A2 L5 A1 | L0 A3 L1 A2
sketch "Sketch10" plane through (0, 0, -14.5) normal (0, 0, -1) x (-0.7478425, 0.6638762, 0)
  circle A0 centre (31.6826, -34.4374) radius 2 projected
  circle A1 centre (16.7809, 33.4776) radius 2 projected
  circle A2 centre (16.7293, -33.2543) radius 2 projected
  circle A3 centre (31.718, 34.8497) radius 2 projected
  line L0 (1.3238, 28.9698) -> (41.2821, 27.1438) projected
  line L1 (41.2821, 27.1438) -> (42.07, 44.385) projected
  line L2 (42.07, 44.385) -> (-7.0508, 34.2824) projected
  arc A4 (-7.0508, 34.2824) -> (-6.3262, -34.4235) centre (0, 0) ccw projected
  line L3 (-6.3262, -34.4235) -> (42.0208, -43.3086) projected
  line L4 (42.0208, -43.3086) -> (41.2821, -27.1438) projected
  line L5 (41.2821, -27.1438) -> (1.3238, -28.9698) projected
  arc A5 (1.3238, 28.9698) -> (1.3238, -28.9698) centre (0, 0) ccw projected
  line L6 (0, 0) -> (-35, 0)
  arc A6 (-7.0508, 34.2824) -> (-6.3262, -34.4235) centre (0, 0) ccw projected
  line L7 (-32.5, -7.5) -> (-32.5, 7.5)
  line L8 (-32.5, 7.5) -> (-37.5, 7.5)
  line L9 (-37.5, 7.5) -> (-37.5, -7.5)
  line L10 (-37.5, -7.5) -> (-32.5, -7.5)
  line L11 (-32.5, -7.5) -> (-37.5, 7.5) construction
  line L12 (-32.5, 7.5) -> (-37.5, -7.5) construction
  line L13 (-25.2452, -28.726) -> (-12.2548, -36.226)
  line L14 (-22.7452, -24.3958) -> (-25.2452, -28.726)
  line L15 (-9.7548, -31.8958) -> (-22.7452, -24.3958)
  line L16 (-12.2548, -36.226) -> (-9.7548, -31.8958)
  line L17 (12.2548, -36.226) -> (25.2452, -28.726)
  line L18 (9.7548, -31.8958) -> (12.2548, -36.226)
  line L19 (22.7452, -24.3958) -> (9.7548, -31.8958)
  line L20 (25.2452, -28.726) -> (22.7452, -24.3958)
  line L21 (37.5, -7.5) -> (37.5, 7.5)
  line L22 (32.5, -7.5) -> (37.5, -7.5)
  line L23 (32.5, 7.5) -> (32.5, -7.5)
  line L24 (37.5, 7.5) -> (32.5, 7.5)
  line L25 (25.2452, 28.726) -> (12.2548, 36.226)
  line L26 (22.7452, 24.3958) -> (25.2452, 28.726)
  line L27 (9.7548, 31.8958) -> (22.7452, 24.3958)
  line L28 (12.2548, 36.226) -> (9.7548, 31.8958)
  line L29 (-12.2548, 36.226) -> (-25.2452, 28.726)
  line L30 (-9.7548, 31.8958) -> (-12.2548, 36.226)
  line L31 (-22.7452, 24.3958) -> (-9.7548, 31.8958)
  line L32 (-25.2452, 28.726) -> (-22.7452, 24.3958)
  point P0 (0, 0)
  point P1 (-10.5983, -33.3568)
  point P2 (-23.5887, -25.8568)
  point P3 (-23.5887, 25.8568)
  point P4 (-10.5983, 33.3568)
  point P5 (-34.187, -7.5)
  point P6 (-34.187, 7.5)
  dimension "d30" = 15
  dimension "d31" = 5
  dimension "d34" = 360
  constraints: 54 end point, 2 midpoint, 2 parallel, 2 perpendicular, 1 horizontal, 1 point on circle, 49 other
  measures "d30" distance of L7.start L7.end
  measures "d31" distance of L8.end L7.end
extrude "Extrusion9" add sketch "Sketch10" against normal up to surface (20.5 mm away) contours A4 L32 L29 L30 | A4 L10 L9 L8 | A4 L16 L13 L14
sketch "Sketch11" plane through (0, 0, -14.5) normal (0, 0, -1) x (-0.7478425, 0.6638762, 0)
  circle A0 centre (31.6826, -34.4374) radius 2 projected
  circle A1 centre (16.7809, 33.4776) radius 2 projected
  circle A2 centre (16.7293, -33.2543) radius 2 projected
  circle A3 centre (31.718, 34.8497) radius 2 projected
  line L0 (1.3238, 28.9698) -> (41.2821, 27.1438) projected
  line L1 (41.2821, 27.1438) -> (42.07, 44.385) projected
  line L2 (42.07, 44.385) -> (-7.0508, 34.2824) projected
  arc A4 (-7.0508, 34.2824) -> (-10.5983, 33.3568) centre (0, 0) ccw projected
  line L3 (-10.5983, 33.3568) -> (-12.2548, 36.226) projected
  line L4 (-12.2548, 36.226) -> (-25.2452, 28.726) projected
  line L5 (-25.2452, 28.726) -> (-23.5887, 25.8568) projected
  arc A5 (-23.5887, 25.8568) -> (-34.187, 7.5) centre (0, 0) ccw projected
  line L6 (-34.187, 7.5) -> (-37.5, 7.5) projected
  line L7 (-37.5, 7.5) -> (-37.5, -7.5) projected
  line L8 (-37.5, -7.5) -> (-34.187, -7.5) projected
  arc A6 (-34.187, -7.5) -> (-23.5887, -25.8568) centre (0, 0) ccw projected
  line L9 (-23.5887, -25.8568) -> (-25.2452, -28.726) projected
  line L10 (-25.2452, -28.726) -> (-12.2548, -36.226) projected
  line L11 (-12.2548, -36.226) -> (-10.5983, -33.3568) projected
  arc A7 (-10.5983, -33.3568) -> (-6.3262, -34.4235) centre (0, 0) ccw projected
  line L12 (-6.3262, -34.4235) -> (42.0208, -43.3086) projected
  line L13 (42.0208, -43.3086) -> (41.2821, -27.1438) projected
  line L14 (41.2821, -27.1438) -> (1.3238, -28.9698) projected
  arc A8 (1.3238, 28.9698) -> (1.3238, -28.9698) centre (0, 0) ccw projected
  line L15 (-37.5, 0) -> (-33.5, 0)
  circle A9 centre (-33.5, 0) radius 2.05
  circle A10 centre (-16.75, -29.0119) radius 2.05
  circle A11 centre (16.75, -29.0119) radius 2.05
  circle A12 centre (33.5, 0) radius 2.05
  circle A13 centre (16.75, 29.0119) radius 2.05
  circle A14 centre (-16.75, 29.0119) radius 2.05
  point P0 (0, 0)
  dimension "d38" = 4
  dimension "d39" = 4.1
  dimension "d42" = 360
  constraints: 6 centre point, 2 end point, 1 coincident, 1 horizontal, 1 midpoint, 13 other
  measures "d38" distance of L15.start L15.end
  measures "d39" diameter of A9
extrude "Extrusion10" cut sketch "Sketch11" against normal blind 5 contours A9 | A10 | A14
fillet "Fillet1" radius 2 6 edges at (30.0706, 17.9097, -4.25) (34.8063, 3.6768, -4.25) (30.5456, -17.0871, -4.25) (20.5874, -28.3047, -4.25) (0.4749, -34.9968, -4.25) (-14.2189, -31.9816, -4.25)
sketch "Sketch12" plane through (0, 0, 1) normal (0, 0, -1) x (-1, 0, 0)
  circle A0 centre (-31.7866, 10.5764) radius 2.05 projected
  circle A1 centre (-25.0527, -22.2399) radius 2.05 projected
  circle A2 centre (6.7339, -32.8162) radius 2.05 projected
  circle A3 centre (46.5558, -4.7204) radius 2 projected
  circle A4 centre (-9.6755, 36.1764) radius 2 projected
  circle A5 centre (34.5876, -13.7627) radius 2 projected
  circle A6 centre (0.5842, 47.1189) radius 2 projected
  line L0 (-18.2423, 22.5437) -> (12.8524, 47.7055) projected
  line L1 (12.8524, 47.7055) -> (1.9955, 61.1223) projected
  line L2 (1.9955, 61.1223) -> (-28.0322, 20.957) projected
  arc A7 (-28.0322, 20.957) -> (-29.2594, 19.2064) centre (0, 0) ccw projected
  arc A8 (-31.5628, 18.4062) -> (-29.2594, 19.2064) centre (-30.9314, 20.3039) ccw projected
  line L3 (-31.5628, 18.4062) -> (-33.2142, 18.9556) projected
  line L4 (-33.2142, 18.9556) -> (-37.9499, 4.7228) projected
  line L5 (-37.9499, 4.7228) -> (-36.2985, 4.1733) projected
  arc A9 (-34.9337, 2.1526) -> (-36.2985, 4.1733) centre (-36.93, 2.2756) ccw projected
  arc A10 (-34.9337, 2.1526) -> (-31.2629, -15.7362) centre (0, 0) ccw projected
  arc A11 (-31.7216, -18.1311) -> (-31.2629, -15.7362) centre (-33.0494, -16.6355) ccw projected
  line L6 (-31.7216, -18.1311) -> (-33.0232, -19.2865) projected
  line L7 (-33.0232, -19.2865) -> (-23.065, -30.5042) projected
  line L8 (-23.065, -30.5042) -> (-21.7635, -29.3488) projected
  arc A12 (-19.3311, -29.1772) -> (-21.7635, -29.3488) centre (-20.4357, -30.8445) ccw projected
  arc A13 (-19.3311, -29.1772) -> (-2.0035, -34.9426) centre (0, 0) ccw projected
  arc A14 (-0.1588, -36.5373) -> (-2.0035, -34.9426) centre (-2.118, -36.9393) ccw projected
  line L9 (-0.1588, -36.5373) -> (0.191, -38.2422) projected
  line L10 (0.191, -38.2422) -> (14.8849, -35.227) projected
  line L11 (14.8849, -35.227) -> (14.535, -33.5221) projected
  arc A15 (15.6026, -31.3298) -> (14.535, -33.5221) centre (16.4942, -33.1201) ccw projected
  arc A16 (15.6026, -31.3298) -> (18.1219, -29.9432) centre (0, 0) ccw projected
  line L12 (18.1219, -29.9432) -> (60.1765, -4.4914) projected
  line L13 (60.1765, -4.4914) -> (48.8927, 7.1069) projected
  line L14 (48.8927, 7.1069) -> (20.2223, -20.786) projected
  arc A17 (-18.2423, 22.5437) -> (20.2223, -20.786) centre (0, 0) ccw projected
  line L15 (-18.2423, 22.5437) -> (12.8524, 47.7055) projected
  line L16 (0, 0) -> (-18.2423, 22.5437)
  circle A18 centre (0, 0) radius 8.075 projected
  arc A19 (-23.2267, 17.3644) -> (15.0153, -24.8101) centre (0, 0) ccw projected
  line L17 (10.3554, -17.1104) -> (15.0153, -24.8101) projected
  arc A20 (10.3554, -17.1104) -> (-16.0184, 11.9754) centre (0, 0) ccw projected
  line L18 (-23.2267, 17.3644) -> (-16.0184, 11.9754) projected
  line L19 (0, 0) -> (20.2223, -20.786)
  line L20 (-18.2423, 22.5437) -> (-22.7144, 28.0702)
  line L21 (1.9955, 61.1223) -> (-28.0322, 20.957) projected
  line L22 (20.2223, -20.786) -> (25.0513, -25.7495)
  line L23 (18.1219, -29.9432) -> (60.1765, -4.4914) projected
  line L24 (-28.0322, 20.957) -> (-16.0184, 11.9754) projected
  line L25 (10.3554, -17.1104) -> (18.1219, -29.9432) projected
  point P0 (13.9464, -14.3352)
  point P1 (-12.5809, 15.5474)
  point P2 (-22.7144, 28.0702)
  constraints: 8 end point, 2 collinear, 2 point on line, 1 perpendicular
extrude "Extrusion11" add sketch "Sketch12" against normal blind 5 contours L16 A20 L18 A17 | A17 L24 L2 L20 | L17 A20 L19 A17 | A17 L22 L12 L25
sketch "Sketch13" plane through (0, 0, 1) normal (0, 0, -1) x (-1, 0, 0)
  circle A0 centre (-31.7866, 10.5764) radius 2.05 projected
  circle A1 centre (-25.0527, -22.2399) radius 2.05 projected
  circle A2 centre (6.7339, -32.8162) radius 2.05 projected
  circle A3 centre (46.5558, -4.7204) radius 2 projected
  circle A4 centre (-9.6755, 36.1764) radius 2 projected
  circle A5 centre (34.5876, -13.7627) radius 2 projected
  circle A6 centre (0.5842, 47.1189) radius 2 projected
  line L0 (-18.2423, 22.5437) -> (12.8524, 47.7055) projected
  line L1 (12.8524, 47.7055) -> (1.9955, 61.1223) projected
  line L2 (1.9955, 61.1223) -> (-28.0322, 20.957) projected
  arc A7 (-28.0322, 20.957) -> (-29.2594, 19.2064) centre (0, 0) ccw projected
  arc A8 (-31.5628, 18.4062) -> (-29.2594, 19.2064) centre (-30.9314, 20.3039) ccw projected
  line L3 (-31.5628, 18.4062) -> (-33.2142, 18.9556) projected
  line L4 (-33.2142, 18.9556) -> (-37.9499, 4.7228) projected
  line L5 (-37.9499, 4.7228) -> (-36.2985, 4.1733) projected
  arc A9 (-34.9337, 2.1526) -> (-36.2985, 4.1733) centre (-36.93, 2.2756) ccw projected
  arc A10 (-34.9337, 2.1526) -> (-31.2629, -15.7362) centre (0, 0) ccw projected
  arc A11 (-31.7216, -18.1311) -> (-31.2629, -15.7362) centre (-33.0494, -16.6355) ccw projected
  line L6 (-31.7216, -18.1311) -> (-33.0232, -19.2865) projected
  line L7 (-33.0232, -19.2865) -> (-23.065, -30.5042) projected
  line L8 (-23.065, -30.5042) -> (-21.7635, -29.3488) projected
  arc A12 (-19.3311, -29.1772) -> (-21.7635, -29.3488) centre (-20.4357, -30.8445) ccw projected
  arc A13 (-19.3311, -29.1772) -> (-2.0035, -34.9426) centre (0, 0) ccw projected
  arc A14 (-0.1588, -36.5373) -> (-2.0035, -34.9426) centre (-2.118, -36.9393) ccw projected
  line L9 (-0.1588, -36.5373) -> (0.191, -38.2422) projected
  line L10 (0.191, -38.2422) -> (14.8849, -35.227) projected
  line L11 (14.8849, -35.227) -> (14.535, -33.5221) projected
  arc A15 (15.6026, -31.3298) -> (14.535, -33.5221) centre (16.4942, -33.1201) ccw projected
  arc A16 (15.6026, -31.3298) -> (18.1219, -29.9432) centre (0, 0) ccw projected
  line L12 (18.1219, -29.9432) -> (60.1765, -4.4914) projected
  line L13 (60.1765, -4.4914) -> (48.8927, 7.1069) projected
  line L14 (48.8927, 7.1069) -> (20.2223, -20.786) projected
  arc A17 (-18.2423, 22.5437) -> (20.2223, -20.786) centre (0, 0) ccw projected
  circle A18 centre (0, 0) radius 8.075 projected
  arc A19 (-23.2267, 17.3644) -> (15.0153, -24.8101) centre (0, 0) ccw projected
  line L15 (18.1219, -29.9432) -> (15.0153, -24.8101) projected
  line L16 (18.1219, -29.9432) -> (25.0513, -25.7495) projected
  line L17 (25.0513, -25.7495) -> (13.9464, -14.3352) projected
  arc A20 (13.9464, -14.3352) -> (-12.5809, 15.5474) centre (0, 0) ccw projected
  line L18 (-12.5809, 15.5474) -> (-22.7144, 28.0702) projected
  line L19 (-22.7144, 28.0702) -> (-28.0322, 20.957) projected
  line L20 (-23.2267, 17.3644) -> (-28.0322, 20.957) projected
  circle A21 centre (0, 0) radius 29
  point P0 (-28.0322, 20.957)
  point P1 (-23.2267, 17.3644)
  point P2 (25.0513, -25.7495)
  point P3 (15.0153, -24.8101)
  dimension "d53" = 58
  constraints: 1 centre point, 1 coincident
  measures "d53" diameter of A21
extrude "Extrusion12" add sketch "Sketch13" along normal blind 5 contours A17 L20 L2 L18 | A17 L17 L12 L15
fillet "Fillet3" radius 2 3 edges at (21.4832, -19.48, 1) (-17.7333, -22.9462, 1) (20.8956, 20.1091, 1)
chamfer "Chamfer2" distance 4 angle 45 18 edges at (-21.5866, -27.8464, 6) (-16.8765, -30.6624, 6) (-14.6961, -32.2445, 6) (-14.71, -34.3746, 6) (11.0499, -33.2099, 6) (20.5765, -28.8494, 6) (22.4143, -29.9265, 6) (0.81, -35.4263, 6) (-0.0161, -37.3897, 6) (34.2856, -7.0354, 6) (35.2726, 3.395, 6) (37.1242, 4.4481, 6) (31.0851, -17.0117, 6) (32.3724, -18.7088, 6) (28.6592, 20.0911, 6) (25.3733, 24.5136, 6) (30.2751, 18.4146, 6) (32.3885, 18.6809, 6)
sketch "Sketch14" plane through (23.065, -30.5042, 2) normal (0.7478425, -0.6638762, 0) x (0, 0, -1)
  line L0 (11.5, 9.55) -> (11.5, 5.45) projected
  line L1 (-4, 11) -> (-4, 4) projected
  line L2 (-4, 7.5) -> (11.5, 7.5)
  circle A0 centre (3.75, 7.5) radius 2
  point P0 (2, 7.5)
  dimension "d60" = 4
  constraints: 3 midpoint, 2 end point, 1 centre point
  measures "d60" diameter of A0
extrude "Extrusion13" cut sketch "Sketch14" against normal blind 12
sketch "Sketch15" plane through (37.9499, 4.7228, 2) normal (0.9488549, 0.3157125, 0) x (0, 0, -1)
  line L0 (-4, 11) -> (-4, 4) projected
  line L1 (11.5, 9.55) -> (11.5, 5.45) projected
  line L2 (11.5, 7.5) -> (-4, 7.5)
  line L3 (-4, -0.575) -> (-4, 15.575) projected
  circle A0 centre (3.75, 7.5) radius 2
  point P0 (2, 7.5)
  dimension "d63" = 4
  constraints: 3 midpoint, 2 end point, 1 centre point
  measures "d63" diameter of A0
extrude "Extrusion14" cut sketch "Sketch15" against normal blind 12
sketch "Sketch16" plane through (-14.8849, -35.227, -14.5) normal (-0.2010124, -0.9795887, 0) x (0.9795887, -0.2010124, 0)
  line L0 (11, 20.5) -> (15, 16.5) projected
  line L1 (11, 20.5) -> (4, 20.5) projected
  line L2 (0, 16.5) -> (4, 20.5) projected
  line L3 (0, 0) -> (0, 16.5) projected
  line L4 (15, 0) -> (0, 0) projected
  line L5 (15, 0) -> (15, 16.5) projected
  line L6 (9.55, 5) -> (5.45, 5) projected
  line L7 (7.5, 5) -> (7.5, 20.5)
  line L8 (11, 20.5) -> (4, 20.5) projected
  circle A0 centre (7.5, 12.75) radius 2
  point P0 (7.5, 14.5)
  dimension "d66" = 4
  constraints: 3 midpoint, 2 end point, 1 centre point
  measures "d66" diameter of A0
extrude "Extrusion15" cut sketch "Sketch16" against normal blind 12 contours A0 L7 | L7 A0
fillet "Fillet4" radius 1.2 2 edges at (-22.6368, -23.2677, -2.2) (20.4784, 25.3069, -2.2)
fillet "Fillet5" radius 6 2 edges at (-13.9464, -14.3352, 3.5) (12.5809, 15.5474, 3.5)
ref_plane "Work Plane6" through (33.0232, -19.2865, -14.5) normal (-0.9795887, 0.2010124, 0) x (0, 0, 1)
sketch "Sketch17" plane through (33.0232, -19.2865, -14.5) normal (-0.9795887, 0.2010124, 0) x (0, 0, 1)
  line L0 (13.5, 25.1195) -> (13.5, -0.6099) projected
  line L1 (16.5, 3.124) -> (16.5, 21.3856) projected
  line L2 (0, 3.124) -> (16.5, 3.124) projected
  line L3 (0, 21.3856) -> (0, 3.124) projected
  line L4 (16.5, 21.3856) -> (0, 21.3856) projected
  line L5 (16.5, 3.124) -> (0, 21.3856)
  line L6 (20.5, 20.3421) -> (16.5, 21.3856) projected
  line L7 (16.5, 21.3856) -> (0, 3.124)
  line L8 (8.25, 11.2548) -> (8.25, 13.2548) construction
  line L9 (13.25, 11.2548) -> (13.25, 13.2548)
  line L10 (3.25, 13.2548) -> (3.25, 11.2548)
  arc A0 (3.25, 11.2548) -> (13.25, 11.2548) centre (8.25, 11.2548) ccw
  arc A1 (13.25, 13.2548) -> (3.25, 13.2548) centre (8.25, 13.2548) ccw
  point P0 (14.5, 12.2548)
  point P1 (8.25, 12.2548)
  dimension "d71" = 1
  dimension "d72" = 10
  constraints: 12 end point, 4 point on circle, 4 tangent, 2 centre point, 2 midpoint, 1 parallel, 1 vertical
  measures "d71" distance of point (8.25, 12.255) L8.end
  measures "d72" diameter of A1
extrude "Extrusion16" cut sketch "Sketch17" along normal blind 12 contours A1 L9 A0 L5 L7 | L7 L5 A1 | L5 L7 A0 L10 A1 | A0 L7 L5
ref_plane "Work Plane7" through (23.065, -30.5042, -14.5) normal (0.3157125, -0.9488549, 0) x (0, 0, 1)
sketch "Sketch18" plane through (23.065, -30.5042, -14.5) normal (0.3157125, -0.9488549, 0) x (0, 0, 1)
  line L0 (16.5, 21.3856) -> (16.5, 3.124) projected
  line L1 (0, 21.3856) -> (16.5, 21.3856) projected
  line L2 (0, 3.124) -> (0, 21.3856) projected
  line L3 (16.5, 3.124) -> (0, 3.124) projected
  line L4 (13.5, 25.1195) -> (13.5, -0.6099) projected
  line L5 (16.5, 21.3856) -> (0, 3.124)
  line L6 (16.5, 3.124) -> (0, 3.124) projected
  line L7 (16.5, 3.124) -> (0, 21.3856)
  line L8 (8.25, 13.2548) -> (8.25, 11.2548) construction
  line L9 (3.25, 13.2548) -> (3.25, 11.2548)
  line L10 (13.25, 11.2548) -> (13.25, 13.2548)
  arc A0 (13.25, 13.2548) -> (3.25, 13.2548) centre (8.25, 13.2548) ccw
  arc A1 (3.25, 11.2548) -> (13.25, 11.2548) centre (8.25, 11.2548) ccw
  point P0 (14.5, 12.2548)
  point P1 (8.25, 12.2548)
  dimension "d75" = 1
  dimension "d76" = 10
  constraints: 12 end point, 4 point on circle, 4 tangent, 2 centre point, 2 midpoint, 1 parallel, 1 vertical
  measures "d75" distance of point (8.25, 12.255) L8.end
  measures "d76" diameter of A1
extrude "Extrusion17" cut sketch "Sketch18" against normal blind 12 contours A0 L10 A1 L7 L5 | L5 L7 A0 | A1 L5 L7 | L7 L5 A1 L9 A0
sketch "Sketch19" plane through (0, 0, 1) normal (0, 0, -1) x (-1, 0, 0)
  arc A0 (-16.9842, 20.9889) -> (18.8277, -19.3525) centre (0, 0) ccw projected
  line L0 (18.8277, -19.3525) -> (17.641, -18.1327) projected
  arc A1 (16.8781, -10.7298) -> (17.641, -18.1327) centre (21.9416, -13.9488) ccw projected
  arc A2 (16.8781, -10.7298) -> (-8.6535, 18.031) centre (0, 0) ccw projected
  arc A3 (-15.9137, 19.666) -> (-8.6535, 18.031) centre (-11.2495, 23.4403) ccw projected
  line L1 (-15.9137, 19.666) -> (-16.9842, 20.9889) projected
  circle A4 centre (0, 0) radius 8.075 projected
  line L2 (0, 0) -> (10.4698, 9.2943)
  circle A5 centre (-25.0527, -22.2399) radius 2.05 projected
  line L3 (0, 0) -> (-25.0527, -22.2399)
  circle A6 centre (10.4698, 9.2943) radius 2.05
  circle A7 centre (-2.8142, 13.7142) radius 2.05
  circle A8 centre (-13.284, 4.42) radius 2.05
  circle A9 centre (-10.4698, -9.2943) radius 2.05
  circle A10 centre (2.8142, -13.7142) radius 2.05
  circle A11 centre (13.284, -4.42) radius 2.05
  dimension "d79" = 14
  dimension "d80" = 4.1
  dimension "d83" = 360
  constraints: 6 centre point, 4 end point, 1 coincident, 1 collinear, 13 other
  measures "d79" distance of L2.start L2.end
  measures "d80" diameter of A6
extrude "Extrusion18" cut sketch "Sketch19" against normal blind 10 contours A9 L3 | L3 A9 | A6 | A7 | A8 | A10 | A11